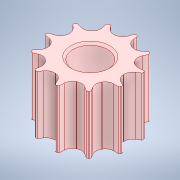
# Autodesk Inventor part: Pulley HTD 3M 11T
Saved by Autodesk Inventor 2022.2 (Build 262287000, 287)
## iProperties
Created: 2019-06-06
Part Number: Pulley HTD 3M 11T
Material: Generic
Description: STEP AP214
Document SubType Name: Modeling
Designer: Jochen
Density: 1 g/cm^3
Appearance: Default
Sending System: PARTsolutions
Title: C:/Users/StangenbergN/Desktop/Steps Zahnriemenräder/K166_HTD-Zahnwellen/17091100.stp
Revision Number: NONE
Autodesk Inventor part; units mm, degrees
ref_plane "YZ Plane" through (0, 0, 0) normal (1, 0, 0) x (0, 1, 0)
ref_plane "XZ Plane" through (0, 0, 0) normal (0, 1, 0) x (-1, 0, 0)
ref_plane "XY Plane" through (0, 0, 0) normal (0, 0, 1) x (1, 0, 0)
sketch "Sketch2" plane through (0, 0, 0) normal (0, 1, 0) x (-1, 0, 0)
  arc A0 (3.5072, -7.2157) -> (3.5837, -7.2232) centre (4.0234, -2.3731) ccw
  arc A1 (3.347, -7.0598) -> (3.5072, -7.2157) centre (3.5264, -7.0357) ccw
  line L0 (3.347, -7.0598) -> (3.283, -6.583)
  arc A2 (3.283, -6.583) -> (2.672, -5.7961) centre (2.3008, -6.715) ccw
  line L1 (2.672, -5.7961) -> (2.6182, -5.7744)
  arc A3 (2.6182, -5.7744) -> (1.632, -5.9162) centre (2.247, -6.6932) ccw
  line L2 (1.632, -5.9162) -> (1.2548, -6.2147)
  arc A4 (1.0313, -6.2155) -> (1.2548, -6.2147) centre (1.1425, -6.0727) ccw
  arc A5 (0.9711, -6.1679) -> (1.0313, -6.2155) centre (4.0234, -2.3731) ccw
  arc A6 (0.9206, -5.9501) -> (0.9711, -6.1679) centre (1.0845, -6.0268) ccw
  line L3 (0.9206, -5.9501) -> (1.1244, -5.5144)
  arc A7 (1.1244, -5.5144) -> (1.0359, -4.5221) centre (0.2269, -5.0944) ccw
  line L4 (1.0359, -4.5221) -> (1.0024, -4.4747)
  arc A8 (1.0024, -4.4747) -> (0.0961, -4.0608) centre (0.1934, -5.0471) ccw
  line L5 (0.0961, -4.0608) -> (-0.3826, -4.1081)
  arc A9 (-0.5711, -3.9879) -> (-0.3826, -4.1081) centre (-0.4003, -3.9279) ccw
  arc A10 (-0.596, -3.9153) -> (-0.5711, -3.9879) centre (4.0234, -2.3731) ccw
  arc A11 (-0.5208, -3.7048) -> (-0.596, -3.9153) centre (-0.4243, -3.8579) ccw
  line L6 (-0.5208, -3.7048) -> (-0.1137, -3.4485)
  arc A12 (-0.1137, -3.4485) -> (0.3483, -2.5658) centre (-0.6417, -2.6099) ccw
  line L7 (0.3483, -2.5658) -> (0.3457, -2.5078)
  arc A13 (0.3457, -2.5078) -> (-0.1929, -1.6697) centre (-0.6443, -2.5519) ccw
  line L8 (-0.1929, -1.6697) -> (-0.6211, -1.4506)
  arc A14 (-0.7148, -1.2476) -> (-0.6211, -1.4506) centre (-0.5387, -1.2895) ccw
  arc A15 (-0.6964, -1.173) -> (-0.7148, -1.2476) centre (4.0234, -2.3731) ccw
  arc A16 (-0.5193, -1.0366) -> (-0.6964, -1.173) centre (-0.521, -1.2176) ccw
  line L9 (-0.5193, -1.0366) -> (-0.0384, -1.0411)
  arc A17 (-0.0384, -1.0411) -> (0.8275, -0.5483) centre (-0.0292, -0.0501) ccw
  line L10 (0.8275, -0.5483) -> (0.8567, -0.4982)
  arc A18 (0.8567, -0.4982) -> (0.8567, 0.4982) centre (0, 0) ccw
  line L11 (0.8567, 0.4982) -> (0.6149, 0.914)
  arc A19 (0.6458, 1.1354) -> (0.6149, 0.914) centre (0.7714, 1.005) ccw
  arc A20 (0.7016, 1.1882) -> (0.6458, 1.1354) centre (4.0234, -2.3731) ccw
  arc A21 (0.9243, 1.2072) -> (0.7016, 1.1882) centre (0.8251, 1.0558) ccw
  line L12 (0.9243, 1.2072) -> (1.3266, 0.9434)
  arc A22 (1.3266, 0.9434) -> (2.3214, 0.8898) centre (1.87, 1.7721) ccw
  line L13 (2.3214, 0.8898) -> (2.3731, 0.9162)
  arc A23 (2.3731, 0.9162) -> (2.9117, 1.7544) centre (1.9217, 1.7985) ccw
  line L14 (2.9117, 1.7544) -> (2.9331, 2.2349)
  arc A24 (3.0788, 2.4044) -> (2.9331, 2.2349) centre (3.1139, 2.2269) ccw
  arc A25 (3.1543, 2.4187) -> (3.0788, 2.4044) centre (4.0234, -2.3731) ccw
  arc A26 (3.3519, 2.3143) -> (3.1543, 2.4187) centre (3.1866, 2.2406) ccw
  line L15 (3.3519, 2.3143) -> (3.5477, 1.8749)
  arc A27 (3.5477, 1.8749) -> (4.3557, 1.292) centre (4.4529, 2.2782) ccw
  line L16 (4.3557, 1.292) -> (4.4134, 1.2863)
  arc A28 (4.4134, 1.2863) -> (5.3197, 1.7002) centre (4.5106, 2.2725) ccw
  line L17 (5.3197, 1.7002) -> (5.5975, 2.0929)
  arc A29 (5.8117, 2.1567) -> (5.5975, 2.0929) centre (5.7452, 1.9883) ccw
  arc A30 (5.8829, 2.1279) -> (5.8117, 2.1567) centre (4.0234, -2.3731) ccw
  arc A31 (5.9927, 1.9332) -> (5.8829, 2.1279) centre (5.8138, 1.9606) ccw
  line L18 (5.9927, 1.9332) -> (5.9199, 1.4577)
  arc A32 (5.9199, 1.4577) -> (6.2844, 0.5305) centre (6.8994, 1.3076) ccw
  line L19 (6.2844, 0.5305) -> (6.3299, 0.4945)
  arc A33 (6.3299, 0.4945) -> (7.3161, 0.3527) centre (6.9449, 1.2716) ccw
  line L20 (7.3161, 0.3527) -> (7.7621, 0.5329)
  arc A34 (7.9768, 0.4708) -> (7.7621, 0.5329) centre (7.8298, 0.3651) ccw
  arc A35 (8.0212, 0.408) -> (7.9768, 0.4708) centre (4.0234, -2.3731) ccw
  arc A36 (8.0083, 0.1849) -> (8.0212, 0.408) centre (7.8726, 0.3047) ccw
  line L21 (8.0083, 0.1849) -> (7.6899, -0.1757)
  arc A37 (7.6899, -0.1757) -> (7.4953, -1.1528) centre (8.4328, -0.8316) ccw
  line L22 (7.4953, -1.1528) -> (7.5141, -1.2077)
  arc A38 (7.5141, -1.2077) -> (8.2671, -1.8601) centre (8.4516, -0.8865) ccw
  line L23 (8.2671, -1.8601) -> (8.7396, -1.9497)
  arc A39 (8.8867, -2.1181) -> (8.7396, -1.9497) centre (8.7059, -2.1275) ccw
  arc A40 (8.8901, -2.1948) -> (8.8867, -2.1181) centre (4.0234, -2.3731) ccw
  arc A41 (8.7586, -2.3756) -> (8.8901, -2.1948) centre (8.7092, -2.2014) ccw
  line L24 (8.7586, -2.3756) -> (8.2958, -2.5068)
  arc A42 (8.2958, -2.5068) -> (7.6039, -3.2236) centre (8.5662, -3.4602) ccw
  line L25 (7.6039, -3.2236) -> (7.59, -3.2799)
  arc A43 (7.59, -3.2799) -> (7.8707, -4.2359) centre (8.5523, -3.5165) ccw
  line L26 (7.8707, -4.2359) -> (8.2199, -4.5667)
  arc A44 (8.2525, -4.7879) -> (8.2199, -4.5667) centre (8.0954, -4.6981) ccw
  arc A45 (8.2139, -4.8543) -> (8.2525, -4.7879) centre (4.0234, -2.3731) ccw
  arc A46 (8.0056, -4.9352) -> (8.2139, -4.8543) centre (8.0582, -4.7621) ccw
  line L27 (8.0056, -4.9352) -> (7.5453, -4.7954)
  arc A47 (7.5453, -4.7954) -> (6.5757, -5.0243) centre (7.2573, -5.7437) ccw
  line L28 (6.5757, -5.0243) -> (6.5336, -5.0642)
  arc A48 (6.5336, -5.0642) -> (6.2529, -6.0202) centre (7.2152, -5.7836) ccw
  line L29 (6.2529, -6.0202) -> (6.3677, -6.4873)
  arc A49 (6.2757, -6.691) -> (6.3677, -6.4873) centre (6.1919, -6.5305) ccw
  arc A50 (6.2072, -6.726) -> (6.2757, -6.691) centre (4.0234, -2.3731) ccw
  arc A51 (5.9882, -6.6814) -> (6.2072, -6.726) centre (6.1261, -6.5642) ccw
  line L30 (5.9882, -6.6814) -> (5.6766, -6.315)
  arc A52 (5.6766, -6.315) -> (4.7371, -5.9833) centre (4.9216, -6.957) ccw
  line L31 (4.7371, -5.9833) -> (4.6801, -5.9941)
  arc A53 (4.6801, -5.9941) -> (3.9272, -6.6466) centre (4.8647, -6.9678) ccw
  line L32 (3.9272, -6.6466) -> (3.7713, -7.1016)
  arc A54 (3.5837, -7.2232) -> (3.7713, -7.1016) centre (3.6, -7.0429) ccw
  circle A55 centre (4.0234, -2.3731) radius 2
  point P0 (4.0234, -2.3731)
  dimension "d1" = 4
  constraints: 110 point on circle, 66 end point, 56 centre point, 1 coincident
  measures "d1" diameter of A55
extrude "Extrusion1" add sketch "Sketch2" along normal blind 6.7
chamfer "Chamfer1" distance 0.25 angle 45 2 edges at (-2.0234, 6.7, -2.3731) (-2.0234, 0, -2.3731)
body "Solid2"
